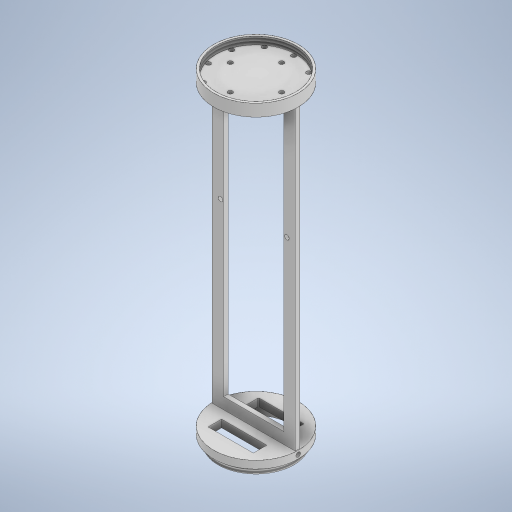
# Autodesk Inventor part: case
Saved by Autodesk Inventor 2023 (Build 270158000, 158)
## iProperties
Created: 2022-07-03
Part Number: case
Material: Generic
Document SubType Name: Modeling
Designer: Administrator
Density: 1 g/cm^3
Appearance: Default
Title: case v1
Author: Administrator
Autodesk Inventor part; units mm, degrees
ref_plane "YZ Plane" through (0, 0, 0) normal (1, 0, 0) x (0, 1, 0)
ref_plane "XZ Plane" through (0, 0, 0) normal (0, 1, 0) x (-1, 0, 0)
ref_plane "XY Plane" through (0, 0, 0) normal (0, 0, 1) x (1, 0, 0)
sketch "Sketch1" plane through (0, 0, 0) normal (0, 0, 1) x (1, 0, 0)
  line L0 (-27.5, 100) -> (27.5, 100)
  line L1 (27.5, 100) -> (27.5, -100)
  line L2 (27.5, -100) -> (-27.5, -100)
  line L3 (-27.5, -100) -> (-27.5, 100)
  line L4 (-20, 92.5) -> (20, 92.5)
  line L5 (20, 92.5) -> (20, -92.5)
  line L6 (20, -92.5) -> (-20, -92.5)
  line L7 (-20, -92.5) -> (-20, 92.5)
  point P0 (0, 0)
  point P1 (0, -100)
  dimension "d0" = 55
  dimension "d1" = 200
  dimension "d2" = 100
  dimension "d3" = 27.5
  dimension "d4" = 185
  dimension "d5" = 40
  dimension "d6" = 20
  dimension "d7" = 92.5
  constraints: 16 end point, 4 parallel, 2 horizontal, 2 perpendicular, 1 midpoint
  measures "d0" distance of L1.end L2.end
  measures "d1" distance of L0.end L1.end
  measures "d2" distance of point (0, -100) point (0, 0)
  measures "d3" distance from line of L3 point (0, 0)
  measures "d4" distance of L6.end L4.start
  measures "d5" distance of L5.end L6.end
  measures "d6" distance from line of L7 point (0, 0)
  measures "d7" distance from line of L4 point (0, 0)
extrude "Extrusion1" add sketch "Sketch1" along normal mid plane 3
sketch "Sketch2" plane through (-27.5, 100, -1.5) normal (0, 1, 0) x (1, 0, 0)
  circle A0 centre (27.5, -1.5) radius 28
  dimension "d10" = 56
  constraints: 1 centre point, 1 coincident
  measures "d10" diameter of A0
extrude "Extrusion2" add sketch "Sketch2" against normal blind 3
sketch "Sketch3" plane through (0, 0, 1.5) normal (0, 0, 1) x (1, 0, 0)
  line L0 (-25, 97) -> (25, 97)
  line L1 (25, 97) -> (25, 17)
  line L2 (25, 17) -> (-25, 17)
  line L3 (-25, 17) -> (-25, 97)
  circle A0 centre (-22, 20) radius 1.5
  circle A1 centre (-22, 94) radius 1.5
  circle A2 centre (22, 20) radius 1.5
  circle A3 centre (22, 94) radius 1.5
  line L4 (-28, 97) -> (28, 97) projected
  point P0 (0, 0)
  dimension "d13" = 80
  dimension "d14" = 50
  dimension "d15" = 25
  dimension "d16" = 3
  dimension "d18" = 3
  dimension "d19" = 3
  dimension "d20" = 3
  dimension "d21" = 44
  dimension "d22" = 44
  dimension "d23" = 22
  dimension "d24" = 22
  dimension "d25" = 74
  dimension "d27" = 74
  dimension "d77" = 0
  dimension "d78" = 3
  dimension "d79" = 3
  constraints: 8 end point, 4 centre point, 2 parallel, 1 horizontal, 1 perpendicular
  measures "d13" distance of L0.end L1.end
  measures "d14" distance of L1.end L2.end
  measures "d15" distance from line of L1 point (0, 0)
  measures "d16" diameter of A0
  measures "d18" diameter of A1
  measures "d19" diameter of A2
  measures "d20" diameter of A3
  measures "d21" distance of A2.centre A0.centre
  measures "d22" distance of A3.centre A1.centre
  measures "d23" horizontal distance of point (0, 0) A1.centre
  measures "d24" horizontal distance of point (0, 0) A0.centre
  measures "d25" distance of A0.centre A1.centre
  measures "d27" distance of A2.centre A3.centre
  measures "d77" distance between parallel lines of L4 L0
  measures "d78" distance from line of L0 A1.centre
  measures "d79" distance from line of L4 A3.centre
extrude "Extrusion3" cut sketch "Sketch3" against normal up to surface (3 mm away) contours A0 | A1 | A2 | A3
sketch "Sketch4" plane through (-27.5, -100, 1.5) normal (0, -1, 0) x (1, 0, 0)
  circle A0 centre (27.5, -1.5) radius 28
  constraints: 1 centre point, 1 coincident
extrude "Extrusion4" add sketch "Sketch4" along normal blind 5
sketch "Sketch5" plane through (0, 0, 0) normal (1, 0, 0) x (0, 1, 0)
  circle A0 centre (-102.5, 0) radius 1.5
  line L0 (-100, 28) -> (-100, -28) projected
  point P0 (0, 0)
  dimension "d33" = 3
  dimension "d34" = 2.5
  constraints: 1 centre point
  measures "d33" diameter of A0
  measures "d34" distance from line of A0.centre L0
extrude "Extrusion5" cut sketch "Sketch5" along normal through all both and the other way through all
thread "Thread1" size "M3x0.5" class "6H" standard "ANSI Metric M Profile" full length
sketch "Sketch6" plane through (0, -105, 0) normal (0, -1, 0) x (1, 0, 0)
  circle A0 centre (0, 0) radius 25
  circle A1 centre (0, 0) radius 22.5
  point P0 (0, 0)
  dimension "d39" = 50
  dimension "d40" = 45
  constraints: 2 centre point, 2 coincident
  measures "d39" diameter of A0
  measures "d40" diameter of A1
extrude "Extrusion6" add sketch "Sketch6" along normal blind 5
thread "Thread2" size "M50x2" class "6g" standard "ANSI Metric M Profile" full length
sketch "Sketch7" plane through (0, -100, 0) normal (0, 1, 0) x (1, 0, 0)
  circle A0 centre (0, 0) radius 22.5 projected
  line L0 (14.7394, 17) -> (-15.2606, 17)
  line L1 (-15.2606, 17) -> (-15.2606, 8)
  line L2 (-15.2606, 8) -> (14.7394, 8)
  line L3 (14.7394, 8) -> (14.7394, 17)
  line L4 (14.7394, -7.5337) -> (-15.2606, -7.5337)
  line L5 (-15.2606, -7.5337) -> (-15.2606, -16.5337)
  line L6 (-15.2606, -16.5337) -> (14.7394, -16.5337)
  line L7 (14.7394, -16.5337) -> (14.7394, -7.5337)
  point P0 (0, 0)
  point P1 (-14.7394, 17)
  point P2 (-15.2606, 16.5337)
  dimension "d45" = 9
  dimension "d46" = 9
  dimension "d47" = 30
  dimension "d48" = 8
  constraints: 16 end point, 4 parallel, 2 horizontal, 2 perpendicular, 2 point on circle, 2 point on line
  measures "d45" distance of L0.end L1.end
  measures "d46" distance of L4.end L5.end
  measures "d47" distance of L5.end L6.end
  measures "d48" distance from line of L2 point (0, 0)
extrude "Extrusion7" cut sketch "Sketch7" against normal blind 10 contours L5 L4 L7 L6 | L3 L2 L1 A0 L0
sketch "Sketch8" plane through (0, 100, 0) normal (0, 1, 0) x (1, 0, 0)
  circle A0 centre (0, -17) radius 1.5
  circle A1 centre (-17, 0) radius 1.5
  circle A2 centre (0, 17) radius 1.5
  circle A3 centre (17, 0) radius 1.5
  point P0 (0, 0)
  dimension "d51" = 3
  dimension "d52" = 3
  dimension "d53" = 3
  dimension "d54" = 3
  dimension "d55" = 34
  dimension "d56" = 34
  dimension "d57" = 17
  dimension "d58" = 17
  constraints: 4 centre point
  measures "d51" diameter of A0
  measures "d52" diameter of A1
  measures "d53" diameter of A2
  measures "d54" diameter of A3
  measures "d55" distance of A2.centre A0.centre
  measures "d56" distance of A1.centre A3.centre
  measures "d57" distance of A3.centre point (0, 0)
  measures "d58" distance of A2.centre point (0, 0)
extrude "Extrusion8" cut sketch "Sketch8" against normal blind 10
sketch "Sketch10" plane through (0, 100, 0) normal (0, 1, 0) x (1, 0, 0)
  circle A0 centre (0, 0) radius 28
  circle A1 centre (0, 0) radius 26.5
  dimension "d80" = 53
  dimension "d81" = 56
  constraints: 2 centre point, 2 coincident
  measures "d80" diameter of A1
  measures "d81" diameter of A0
extrude "Extrusion10" add sketch "Sketch10" along normal blind 5
thread "Thread3" size "M55x2" class "6H" standard "ANSI Metric M Profile" full length
sketch "Sketch11" plane through (0, 100, 0) normal (0, 1, 0) x (1, 0, 0)
  circle A0 centre (0, 0) radius 25 projected
  circle A1 centre (0, 25) radius 1.5
  point P0 (0, 0)
  dimension "d86" = 3
  constraints: 1 centre point, 1 vertical alignment, 1 other
  measures "d86" diameter of A1
extrude "Extrusion11" cut sketch "Sketch11" against normal up to surface (3 mm away) contours A1 A0 | A0 A1 picked at (-0.0591, 24.5002) picked at (0.0534, 25.4938)
pattern_circular "Circular Pattern1" count 10 over 360 about axis through (0, 100, 0) along (0, -1, 0) of "Extrusion11"
body "Solid1"
